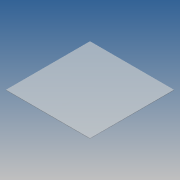
# Autodesk Inventor part: plinth
Saved by Autodesk Inventor 2014 SP1 (Build 180222100, 222)
## iProperties
Created: 2014-03-11
Part Number: plinth
Material: Glass
Document SubType Name: Modeling
Designer: Dave
Density: 2.18 g/cm^3
Appearance: Clear
Mass: 9837.25 g
Surface Area: 18240 cm^2
Volume: 4512.5 cm^3
Author: Dave
Autodesk Inventor part; units mm, degrees
ref_plane "YZ Plane" through (0, 0, 0) normal (1, 0, 0) x (0, 1, 0)
ref_plane "XZ Plane" through (0, 0, 0) normal (0, 1, 0) x (-1, 0, 0)
ref_plane "XY Plane" through (0, 0, 0) normal (0, 0, 1) x (1, 0, 0)
sketch "Sketch1" plane through (0, 0, 0) normal (0, 1, 0) x (-1, 0, 0)
  line L0 (0, 0) -> (950, 0)
  line L1 (950, 0) -> (950, 950)
  line L2 (950, 950) -> (0, 950)
  line L3 (0, 950) -> (0, 0)
  dimension "d0" = 950
  dimension "d1" = 950
  constraints: 8 end point, 2 parallel, 1 horizontal, 1 perpendicular
  measures "d0" distance of L2.end L1.end
  measures "d1" distance of L2.end L0.start
extrude "Extrusion1" add sketch "Sketch1" along normal blind 5
body "Solid1"
